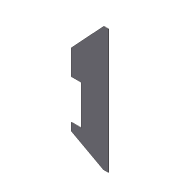
# Autodesk Inventor part: Conveyor_Frame_BottomStabilizerPlate
Saved by Autodesk Inventor 2012 (Build 160160000, 160)
## iProperties
Created: 2012-01-09
Part Number: Conveyor_Frame_BottomStabilizerPlate
Material: Aluminum-6061
Document SubType Name: Modeling
Designer: JesseK
Density: 2.71 g/cm^3
Mass: 762.585 g
Surface Area: 1822.93 cm^2
Volume: 281.397 cm^3
Author: JesseK
Autodesk Inventor part; units mm, degrees
ref_plane "YZ Plane" through (0, 0, 0) normal (1, 0, 0) x (0, 1, 0)
ref_plane "XZ Plane" through (0, 0, 0) normal (0, 1, 0) x (-1, 0, 0)
ref_plane "XY Plane" through (0, 0, 0) normal (0, 0, 1) x (1, 0, 0)
sketch "Sketch1" plane through (0, 0, 0) normal (0, 0, 1) x (1, 0, 0)
  line L0 (0, 0) -> (190.5, 0)
  line L1 (190.5, 0) -> (190.5, 635)
  line L2 (190.5, 635) -> (0, 635)
  line L3 (0, 635) -> (0, 0)
  dimension "d0" = 190.5
  dimension "d1" = 635
  constraints: 8 end point, 2 parallel, 1 horizontal, 1 perpendicular
  measures "d0" distance of L1.end L2.end
  measures "d1" distance of L2.end L0.start
extrude "Extrusion1" add sketch "Sketch1" along normal blind 3.175
sketch "Sketch2" plane through (0, 0, 3.175) normal (0, 0, 1) x (1, 0, 0)
  line L0 (0, 0) -> (0, 635) projected
  line L1 (190.5, 0) -> (0, 0) projected
  line L2 (165.1, 0) -> (0, 0)
  line L3 (0, 88.9) -> (165.1, 0)
  line L4 (0, 635) -> (190.5, 635) projected
  line L5 (165.1, 635) -> (0, 635)
  line L6 (0, 457.2) -> (165.1, 635)
  line L7 (0, 457.2) -> (0, 635)
  line L8 (165.1, 635) -> (165.1, 0) construction
  line L9 (190.5, 635) -> (190.5, 0) projected
  dimension "d5" = 88.9
  dimension "d8" = 177.8
  dimension "d9" = 25.4
  constraints: 12 end point, 4 point on line, 2 vertical, 1 collinear, 1 horizontal
  measures "d5" distance of L0.start L3.start
  measures "d8" distance of L0.end L6.start
  measures "d9" distance from line of L9 L2.start
extrude "Extrusion2" cut sketch "Sketch2" against normal up to next contours L0 L3 L1 | L0 L4 L6
sketch "Sketch4" plane through (0, 0, 3.175) normal (0, 0, 1) x (1, 0, 0)
  line L0 (0, 88.9) -> (0, 457.2) projected
  line L1 (0, 330.2) -> (50.8, 330.2)
  line L2 (50.8, 330.2) -> (50.8, 127)
  line L3 (50.8, 127) -> (0, 127)
  line L4 (0, 127) -> (0, 330.2)
  line L5 (165.1, 635) -> (50.8, 635) construction
  line L6 (50.8, 635) -> (50.8, 330.2) construction
  line L7 (50.8, 127) -> (50.8, 0) construction
  line L8 (50.8, 0) -> (165.1, 0) construction
  point P0 (0, 0)
  dimension "d17" = 203.2
  dimension "d18" = 50.8
  dimension "d21" = 127
  constraints: 16 end point, 3 horizontal, 2 parallel, 2 vertical, 1 perpendicular, 1 point on line
  measures "d17" distance of L1.end L2.end
  measures "d18" distance of L1.start L1.end
  measures "d21" distance of L2.end L7.end
extrude "Extrusion4" cut sketch "Sketch4" against normal through all
body "Solid1"
